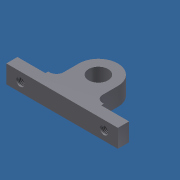
# Autodesk Inventor part: MANCAL DA BETONEIRA(26)
Saved by Autodesk Inventor 2012 SP1 (Build 160190100, 190)
## iProperties
Created: 2012-07-23
Part Number: MANCAL DA BETONEIRA(26)
Material: Carbon Steel
Document SubType Name: Modeling
Designer: bruno.silveira
Mass: 153.953 g
Surface Area: 72.7469 cm^2
Volume: 19.562 cm^3
Density: 7.87 g/cm^3
Author: bruno.silveira
Autodesk Inventor part; units mm, degrees
ref_plane "YZ Plane" through (0, 0, 0) normal (1, 0, 0) x (0, 1, 0)
ref_plane "XZ Plane" through (0, 0, 0) normal (0, 1, 0) x (-1, 0, 0)
ref_plane "XY Plane" through (0, 0, 0) normal (0, 0, 1) x (1, 0, 0)
sketch "Sketch1" plane through (0, 0, 0) normal (0, 0, 1) x (1, 0, 0)
  line L0 (0, 0) -> (80, 0)
  line L1 (80, 0) -> (80, 40)
  line L2 (80, 40) -> (0, 40)
  line L3 (0, 40) -> (0, 0)
  dimension "d0" = 80
  dimension "d1" = 40
  constraints: 8 end point, 2 parallel, 1 horizontal, 1 perpendicular
  measures "d0" distance of L0.start L0.end
  measures "d1" distance of L2.end L0.start
extrude "Extrusion1" add sketch "Sketch1" along normal blind 13
sketch "Sketch2" plane through (0, 0, 13) normal (0, 0, 1) x (1, 0, 0)
  line L0 (80, 0) -> (0, 0) projected
  line L1 (80, 40) -> (80, 0) projected
  point P0 (40, 26)
  dimension "d4" = 26
  dimension "d5" = 40
  measures "d4" distance from line of L0 point (40, 26)
  measures "d5" distance from line of L1 point (40, 26)
hole "Hole1" at (40, 26, 13) direction (0, 0, -1) diameter 14 depth 13 tip angle 118
sketch "Sketch3" plane through (0, 0, 13) normal (0, 0, 1) x (1, 0, 0)
  circle A0 centre (40, 26) radius 7 projected
  line L0 (0, 0) -> (0, 40) projected
  line L1 (80, 0) -> (0, 0) projected
  line L2 (80, 40) -> (80, 0) projected
  line L3 (0, 40) -> (80, 40) projected
  arc A1 (54, 26) -> (26, 26) centre (40, 26) ccw
  line L4 (54, 26) -> (54, 10)
  line L5 (26, 26) -> (26, 10)
  line L6 (0, 10) -> (26, 10)
  line L7 (54, 10) -> (80, 10)
  dimension "d14" = 10
  dimension "d15" = 10
  dimension "d16" = 26
  constraints: 8 end point, 6 perpendicular, 2 point on circle, 2 point on line, 2 tangent, 1 centre point, 1 coincident
  measures "d14" distance between parallel lines of L1 L7
  measures "d15" distance between parallel lines of L1 L6
  measures "d16" distance between parallel lines of L0 L5
extrude "Extrusion2" cut sketch "Sketch3" against normal blind 13 contours L0 L3 A1 L5 L6 | L7 L4 A1 L3 L2
sketch "Sketch6" plane through (54, 10, 13) normal (0, 1, 0) x (1, 0, 0)
  line L0 (0, 13) -> (26, 13) projected
  line L1 (0, 0) -> (0, 13) projected
  line L2 (26, 0) -> (0, 0) projected
  line L3 (26, 13) -> (26, 0) projected
  line L4 (-54, 13) -> (-28, 13) projected
  line L5 (-54, 0) -> (-54, 13) projected
  line L6 (-28, 0) -> (-54, 0) projected
  line L7 (-28, 0) -> (-28, 13) projected
  line L8 (-34, 13) -> (-34, 0)
  line L9 (6, 13) -> (6, 0)
  point P0 (-54, 13)
  dimension "d36" = 40
  dimension "d37" = 6
  constraints: 4 end point, 4 point on line, 2 perpendicular
  measures "d36" distance between parallel lines of L9 L8
  measures "d37" distance between parallel lines of L1 L9
extrude "Extrusion4" cut sketch "Sketch6" against normal blind 2 contours L0 L3 L2 L9 | L4 L8 L6 L5
sketch "Sketch7" plane through (54, 8, 13) normal (0, 1, 0) x (1, 0, 0)
  line L0 (-54, 13) -> (-34, 13) projected
  line L1 (-54, 0) -> (-54, 13) projected
  line L2 (6, 13) -> (6, 0) projected
  line L3 (26, 0) -> (6, 0) projected
  line L4 (26, 13) -> (26, 0) projected
  line L5 (6, 13) -> (26, 13) projected
  point P0 (-44, 6.5)
  point P1 (16, 6.5)
  dimension "d40" = 60
  dimension "d41" = 6.5
  dimension "d42" = 10
  measures "d40" distance of point (-44, 6.5) point (16, 6.5)
  measures "d41" distance from line of L0 point (-44, 6.5)
  measures "d42" distance from line of L1 point (-44, 6.5)
hole "Hole3" at (10, 8, 6.5) at (70, 8, 6.5) direction (0, -1, 0) diameter 4.917 depth 8 tip angle 118 thread size "M6x1" class "6H" standard "ANSI Metric M Profile"
chamfer "Chamfer1" distance 0.5 angle 45 4 edges at (10, 8, 4.0415) (70, 8, 4.0415) (10, 0, 4.0415) (70, 0, 4.0415)
fillet "Fillet2" radius 5 2 edges at (26, 10, 6.5) (54, 10, 6.5)
body "Solid1"
